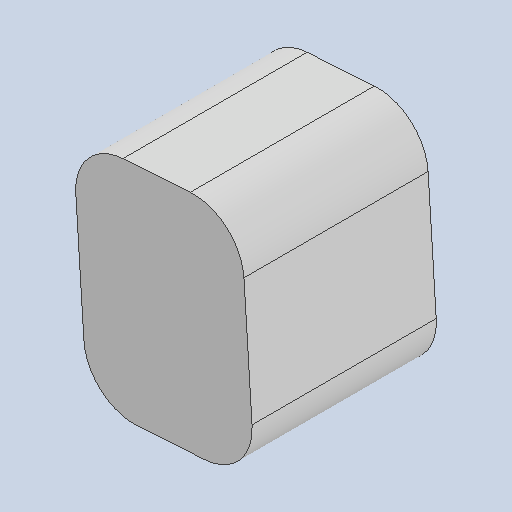
# Autodesk Inventor part: wspornik
Saved by Autodesk Inventor 2023 (Build 270158000, 158)
## iProperties
Created: 2023-01-29
Part Number: wspornik
Material: Generic
Document SubType Name: Modeling
Designer: Kamil
Density: 1 g/cm^3
Appearance: Default
Mass: 37.0634 g
Surface Area: 63.4437 cm^2
Volume: 37.0634 cm^3
Author: Kamil
Autodesk Inventor part; units mm, degrees
ref_plane "YZ Plane" through (0, 0, 0) normal (1, 0, 0) x (0, 1, 0)
ref_plane "XZ Plane" through (0, 0, 0) normal (0, 1, 0) x (-1, 0, 0)
sketch "Sketch1" plane through (0, 0, 0) normal (0, 0, 1) x (1, 0, 0)
  circle A0 centre (9.0867, 110.4972) radius 1.6 projected
  arc A1 (10.396, 90.5401) -> (7.7775, 130.4543) centre (9.0867, 110.4972) ccw projected
  line L0 (-242.3149, 114.047) -> (7.7775, 130.4543) projected
  line L1 (-239.6964, 74.1328) -> (-242.3149, 114.047) projected
  line L2 (10.396, 90.5401) -> (-239.6964, 74.1328) projected
  circle A2 centre (9.0867, 110.4972) radius 20
  line L3 (-242.3149, 114.047) -> (-212.3793, 116.0109)
  line L4 (-212.3793, 116.0109) -> (-209.7607, 76.0967)
  point P0 (0, 0)
  dimension "d0" = 30
  constraints: 4 end point, 2 point on line, 1 centre point, 1 coincident, 1 concentric, 1 perpendicular
  measures "d0" distance of L0.start L3.end
ref_plane "Work Plane1" through (-89.0919, -102.1665, 32.7858) normal (0, 0, -1) x (0, 1, 0)
extrude "Extrusion1" add sketch "Sketch1" along normal up to surface (32.7858 mm away) contours L2 L1 L0 L4
fillet "Fillet1" radius 9 4 edges at (-209.7607, 76.0967, 16.3929) (-239.6964, 74.1328, 16.3929) (-212.3793, 116.0109, 16.3929) (-242.3149, 114.047, 16.3929)
body "Solid1"
